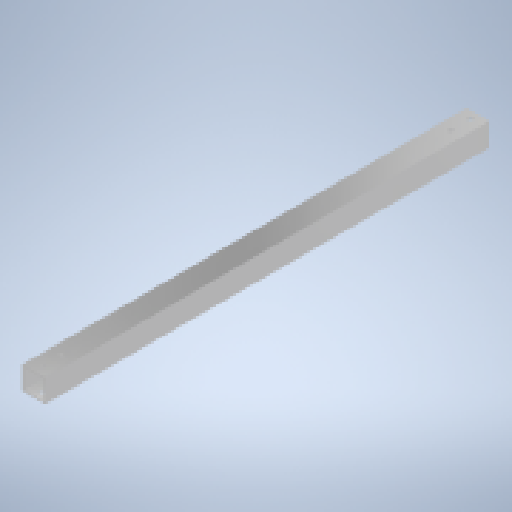
# Autodesk Inventor part: pipe_elbow2hand
Saved by Autodesk Inventor 2026.1 (Build 301233020, 233B)
## iProperties
Created: 2026-02-01
Part Number: pipe_elbow2hand
Material: アルミニウム 6061
Document SubType Name: Modeling
Designer: hibik
Density: 2.7 g/cm^3
Appearance: アルミニウム - フラット
Author: hibik
Autodesk Inventor part; units mm, degrees
ref_plane "YZ Plane" through (0, 0, 0) normal (1, 0, 0) x (0, 1, 0)
ref_plane "XZ Plane" through (0, 0, 0) normal (0, 1, 0) x (-1, 0, 0)
ref_plane "XY Plane" through (0, 0, 0) normal (0, 0, 1) x (1, 0, 0)
sketch "スケッチ1" plane through (0, 0, 0) normal (0, 0, 1) x (1, 0, 0)
  line L0 (-7.5, 7.5) -> (7.5, 7.5)
  line L1 (7.5, 7.5) -> (7.5, -7.5)
  line L2 (7.5, -7.5) -> (-7.5, -7.5)
  line L3 (-7.5, -7.5) -> (-7.5, 7.5)
  point P0 (0, 0)
  point P1 (-7.5, 0)
  point P2 (0, 7.5)
  dimension "d0" = 15
  dimension "d1" = 15
  constraints: 8 end point, 2 midpoint, 2 parallel, 1 horizontal, 1 horizontal alignment, 1 perpendicular, 1 vertical alignment
  measures "d0" distance of L1.end L2.end
  measures "d1" distance of L0.end L1.end
extrude "押し出し1" add sketch "スケッチ1" along normal blind 290
shell "シェル1" thickness 1 removed faces 2 at (-2.5, -2.5, 0) at (-2.5, -2.5, 290)
sketch "スケッチ2" plane through (-7.5, 7.5, 0) normal (0, 1, 0) x (1, 0, 0)
  circle A0 centre (7.5, -5) radius 1.6
  circle A1 centre (7.5, -18) radius 1.6
  circle A2 centre (7.5, -272) radius 1.6
  circle A3 centre (7.5, -285) radius 1.6
  line L0 (15, 0) -> (0, 0) projected
  line L1 (15, -290) -> (0, -290) projected
  point P0 (7.5, 0)
  point P1 (7.5, 0)
  point P2 (7.5, 0)
  dimension "d5" = 3.2
  dimension "d6" = 3.2
  dimension "d7" = 3.2
  dimension "d8" = 3.2
  dimension "d9" = 5
  dimension "d10" = 13
  dimension "d11" = 5
  dimension "d12" = 13
  constraints: 4 centre point, 4 vertical alignment, 2 midpoint
  measures "d5" diameter of A0
  measures "d6" diameter of A1
  measures "d7" diameter of A2
  measures "d8" diameter of A3
  measures "d9" distance from line of A3.centre L1
  measures "d10" distance of A2.centre A3.centre
  measures "d11" distance of point (7.5, 0) A0.centre
  measures "d12" distance of A1.centre A0.centre
extrude "押し出し2" cut sketch "スケッチ2" against normal through all
